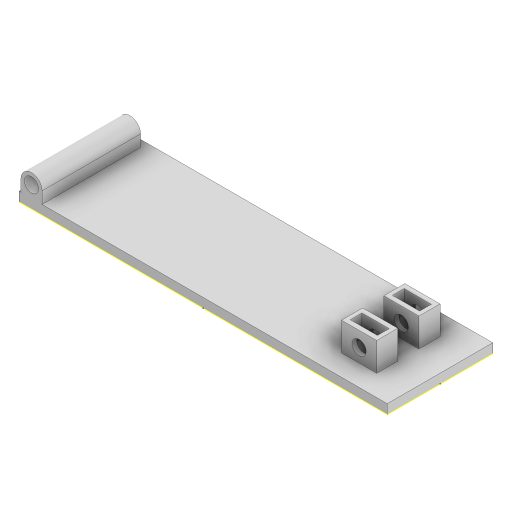
# Autodesk Inventor part: vrata
Saved by Autodesk Inventor 2023.3 (Build 273359000, 359)
## iProperties
Created: 2025-03-15
Part Number: vrata
Material: Generic
Document SubType Name: Modeling
Designer: David Zindović
Density: 1 g/cm^3
Appearance: Default
Author: David Zindović
Autodesk Inventor part; units mm, degrees
ref_plane "YZ Plane" through (0, 0, 0) normal (1, 0, 0) x (0, 1, 0)
ref_plane "XZ Plane" through (0, 0, 0) normal (0, 1, 0) x (-1, 0, 0)
ref_plane "XY Plane" through (0, 0, 0) normal (0, 0, 1) x (1, 0, 0)
sketch "Sketch1" plane through (0, 0, 0) normal (0, 0, 1) x (1, 0, 0)
  line L0 (-39.25, 1) -> (39.25, 1)
  line L1 (39.25, 1) -> (39.25, -1)
  line L2 (39.25, -1) -> (-39.25, -1)
  line L3 (-39.25, -1) -> (-39.25, 1)
  circle A0 centre (-36.63, 3.5) radius 1.5
  circle A1 centre (28.75, 3.875) radius 1.5
  line L4 (39.25, 6.75) -> (38, 6.75)
  line L5 (38, 6.75) -> (38, 26.75)
  line L6 (38, 26.75) -> (-38, 26.75)
  line L7 (-38, 26.75) -> (-38, 6.75)
  line L8 (-38, 6.75) -> (-39.25, 6.75)
  line L9 (-39.25, 6.75) -> (-39.25, 1)
  line L10 (-39.25, 1) -> (39.25, 1)
  line L11 (39.25, 6.75) -> (39.25, 1)
  line L12 (-34.38, 1) -> (-38.88, 1)
  line L13 (-38.88, 1) -> (-38.88, 3.5)
  line L14 (-38.88, 3.5) -> (-34.38, 3.5)
  line L15 (-34.38, 3.5) -> (-34.38, 1)
  arc A2 (-34.38, 3.5) -> (-38.88, 3.5) centre (-36.63, 3.5) ccw
  line L16 (31, 1) -> (26.5, 1)
  line L17 (26.5, 1) -> (26.5, 3.875)
  line L18 (26.5, 3.875) -> (31, 3.875)
  line L19 (31, 3.875) -> (31, 1)
  arc A3 (31, 3.875) -> (26.5, 3.875) centre (28.75, 3.875) ccw
  line L20 (31.5, 5.4627) -> (31.5, 2.2873)
  line L21 (31.5, 2.2873) -> (28.75, 0.6996)
  line L22 (28.75, 0.6996) -> (26, 2.2873)
  line L23 (26, 2.2873) -> (26, 5.4627)
  line L24 (26, 5.4627) -> (28.75, 7.0504)
  line L25 (28.75, 7.0504) -> (31.5, 5.4627)
  line L26 (32.5, 1) -> (25, 1)
  line L27 (25, 1) -> (25, 7.0504)
  line L28 (25, 7.0504) -> (32.5, 7.0504)
  line L29 (32.5, 7.0504) -> (32.5, 1)
  point P0 (0, 0)
  point P1 (0, 1)
  point P2 (39.25, 0)
  point P3 (0, 35)
  point P4 (28.75, 7.0504)
  dimension "d0" = 2
  dimension "d1" = 78.5
  dimension "d4" = 2.62
  dimension "d5" = 2.5
  dimension "d6" = 3
  dimension "d7" = 4.5
  dimension "d8" = 2.875
  dimension "d9" = 10.5
  dimension "d10" = 3
  dimension "d11" = 4.5
  dimension "d12" = 5.5
  dimension "d13" = 7.5
  dimension "d14" = 0
  constraints: 60 end point, 8 parallel, 5 coincident, 5 midpoint, 4 centre point, 4 horizontal, 4 perpendicular, 4 point on circle, 3 point on line, 3 vertical alignment, 2 vertical, 1 horizontal alignment, 13 other
  measures "d0" distance of L0.end L1.end
  measures "d1" distance of L0.start L0.end
  measures "d4" distance from line of L9 A0.centre
  measures "d5" distance from line of L0 A0.centre
  measures "d6" diameter of A0
  measures "d7" distance between parallel lines of L15 L13
  measures "d8" distance from line of L0 A1.centre
  measures "d9" distance from line of L11 A1.centre
  measures "d10" diameter of A1
  measures "d11" distance between parallel lines of L19 L17
  measures "d12" distance between parallel lines of L23 L20
  measures "d13" distance between parallel lines of L29 L27
  measures "d14" distance from line of L24.end L28
extrude "Extrusion1" add sketch "Sketch1" along normal blind 22.5 contours L0 L22 L21 L1 L2 L3 | L13 L14 A0 L15 L0 | A2 L14 A0 | L27 L28 L24 L23 L22 L17 L0 | L17 L22 L0 | L0 L19 L21 L20 L25 L28 L29 | L22 L17 L18 A1 L19 L21 L0 | L0 L21 L22 | L22 L23 L24 L25 L20 L21 L19 A3 L17 | L0 L21 L19 | A3 L18 A1
sketch "Sketch2" plane through (39.25, -1, 0) normal (1, 0, 0) x (0, 0, -1)
  line L0 (-22.5, 0) -> (-22.5, 2) projected
  line L1 (0, 8.0504) -> (-22.5, 8.0504) projected
  line L2 (-22.5, 2) -> (-18, 2)
  line L3 (-18, 2) -> (-18, 8.0504)
  line L4 (-18, 8.0504) -> (-22.5, 8.0504)
  line L5 (-22.5, 8.0504) -> (-22.5, 2)
  line L6 (-18, 2) -> (-13.5, 2)
  line L7 (-13.5, 2) -> (-13.5, 8.0504)
  line L8 (-13.5, 8.0504) -> (-18, 8.0504)
  line L9 (-18, 8.0504) -> (-18, 2)
  line L10 (0, 2) -> (-22.5, 2) projected
  line L11 (-4.5, 2) -> (-9, 2)
  line L12 (-9, 2) -> (-9, 8.0504)
  line L13 (-9, 8.0504) -> (-4.5, 8.0504)
  line L14 (-4.5, 8.0504) -> (-4.5, 2)
  line L15 (0, 2) -> (-4.5, 2)
  line L16 (-4.5, 2) -> (-4.5, 8.0504)
  line L17 (-4.5, 8.0504) -> (0, 8.0504)
  line L18 (0, 8.0504) -> (0, 2)
  line L19 (-9, 8.0504) -> (-13.5, 8.0504)
  line L20 (-13.5, 8.0504) -> (-13.5, 2)
  line L21 (-13.5, 2) -> (-9, 2)
  line L22 (-9, 2) -> (-9, 8.0504)
  point P0 (0, 1)
  dimension "d15" = 4.5
  dimension "d16" = 4.5
  dimension "d17" = 4.5
  dimension "d18" = 4.5
  constraints: 40 end point, 10 parallel, 5 horizontal, 5 perpendicular, 4 point on line
  measures "d15" distance between parallel lines of L3 L7
  measures "d16" distance between parallel lines of L5 L3
  measures "d17" distance between parallel lines of L14 L12
  measures "d18" distance between parallel lines of L7 L12
extrude "Extrusion2" cut sketch "Sketch2" against normal up to surface (14.25 mm away) contours L18 L10 L14 L1 | L12 L10 L7 L1 | L3 L2 L5 L1
sketch "Sketch3" plane through (25, 7.0504, 18) normal (0, 1, 0) x (1, 0, 0)
  line L0 (6.65, 1) -> (0.85, 1)
  line L1 (0.85, 1) -> (0.85, 3.5)
  line L2 (0.85, 3.5) -> (6.65, 3.5)
  line L3 (6.65, 3.5) -> (6.65, 1)
  line L4 (0, 0) -> (7.5, 0) projected
  line L5 (7.5, 4.5) -> (7.5, 0) projected
  line L6 (6.65, 10) -> (0.85, 10)
  line L7 (0.85, 10) -> (0.85, 12.5)
  line L8 (0.85, 12.5) -> (6.65, 12.5)
  line L9 (6.65, 12.5) -> (6.65, 10)
  line L10 (0, 9) -> (7.5, 9) projected
  line L11 (7.5, 13.5) -> (7.5, 9) projected
  point P0 (-25, 18)
  point P1 (3.75, 1)
  point P2 (3.75, 0)
  point P3 (6.65, 2.25)
  point P4 (7.5, 2.25)
  point P5 (3.75, 10)
  point P6 (3.75, 9)
  point P7 (6.65, 11.25)
  point P8 (7.5, 11.25)
  dimension "d21" = 5.8
  dimension "d22" = 2.5
  dimension "d23" = 5.8
  dimension "d24" = 2.5
  constraints: 16 end point, 8 midpoint, 4 parallel, 2 horizontal, 2 horizontal alignment, 2 perpendicular, 2 vertical alignment
  measures "d21" distance of L1.end L2.end
  measures "d22" distance of L0.end L1.end
  measures "d23" distance of L6.start L6.end
  measures "d24" distance of L6.end L7.end
extrude "Extrusion3" cut sketch "Sketch3" against normal blind 6.351
sketch "Sketch4" plane through (25.85, 7.0504, 5.5) normal (0, 0, 1) x (1, 0, 0)
  circle A0 centre (2.9, -3.1754) radius 1.5 projected
  line L0 (0, 0) -> (5.8, 0) projected
  line L1 (0, 0) -> (0, -6.351) projected
  line L2 (0, -6.351) -> (5.8, -6.351) projected
  line L3 (5.8, 0) -> (5.8, -6.351) projected
  line L4 (2.9, -6.351) -> (0, -4.6767)
  line L5 (0.1499, -4.7632) -> (0.1499, -1.5876)
  line L6 (0.1499, -1.5876) -> (2.9, 0.0001)
  line L7 (2.9, 0.0001) -> (5.6501, -1.5876)
  line L8 (5.6501, -1.5876) -> (5.6501, -4.7632)
  line L9 (5.8, -4.6767) -> (2.9, -6.351)
  point P0 (-25.85, -7.0504)
  constraints: 12 end point, 4 point on line, 1 coincident, 1 midpoint, 1 vertical alignment, 13 other
extrude "Extrusion4" add sketch "Sketch4" along normal up to surface (2.5 mm away) contours L4 L2 L1 | L3 L2 L9
ref_plane "Work Plane1" through (25, 7.0504, 11.25) normal (0, 0, 1) x (1, 0, 0)
mirror "Mirror1" about plane through (25, 7.0504, 11.25) normal (0, 0, 1) of "Extrusion4"
sketch "Sketch5" plane through (-39.25, -1, 0) normal (0, -1, 0) x (1, 0, 0)
  line L0 (6.1251, 17.7549) -> (72.3749, 17.7549) construction
  line L1 (72.3749, 17.7549) -> (72.3749, 4.7451) construction
  line L2 (72.3749, 4.7451) -> (6.1251, 4.7451) construction
  line L3 (6.1251, 4.7451) -> (6.1251, 17.7549) construction
  line L4 (0, 22.5) -> (78.5, 22.5) projected
  line L5 (78.5, 0) -> (78.5, 22.5) projected
  point P0 (39.25, 0)
  point P1 (39.25, 17.7549)
  point P2 (39.25, 22.5)
  point P3 (72.3749, 11.25)
  point P4 (78.5, 11.25)
  constraints: 4 midpoint, 1 horizontal alignment, 1 vertical, 1 vertical alignment, 2 other
sketch "Sketch6" plane through (-39.25, -1, 0) normal (-1, 0, 0) x (0, 0, 1)
  line L0 (0, 0) -> (0, 2) projected
  line L1 (0, 6.75) -> (22.5, 6.75) projected
  line L2 (0, 2) -> (1.5, 2)
  line L3 (1.5, 2) -> (1.5, 6.75)
  line L4 (1.5, 6.75) -> (0, 6.75)
  line L5 (0, 6.75) -> (0, 2)
  point P0 (0, 1)
  dimension "d30" = 1.5
  constraints: 8 end point, 2 parallel, 1 horizontal, 1 perpendicular, 1 point on line
  measures "d30" distance of L0.end L2.end
extrude "Extrusion5" cut sketch "Sketch6" against normal blind 10
equation "\"d11\" = d7"
equation "\"d17\" = d15"
equation "\"d18\" = d16"
equation "\"d23\" = d21"
equation "\"d24\" = d22"
body "Solid1"
